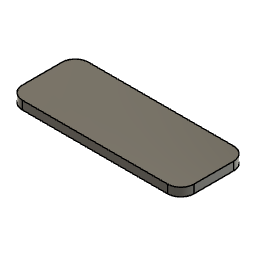
Locker Sign (Autodesk Fusion 360 design; units mm, degrees)
Autodesk Fusion 360 part; units mm, degrees
note: some values were not read from the file. Set by a fixed rule: which sketch regions a step uses.
sketch "Sketch1" plane through (0, 0, 0) normal (0, 1, 0) x (1, 0, 0)
  line L0 (30, 50) -> (140, 50)
  line L1 (150, 40) -> (150, 10)
  line L2 (140, 0) -> (30, 0)
  line L3 (20, 10) -> (20, 40)
  arc A0 (150, 40) -> (140, 50) centre (140, 40) ccw
  arc A1 (140, 0) -> (150, 10) centre (140, 10) ccw
  arc A2 (30, 50) -> (20, 40) centre (30, 40) ccw
  arc A3 (20, 10) -> (30, 0) centre (30, 10) ccw
  point P0 (20, 50)
  point P1 (150, 50)
  point P2 (20, 0)
  dimension "d1" = 130
  dimension "d2" = 50
  dimension "d7" = 10
  dimension "d8" = 10
  dimension "d9" = 10
  dimension "d10" = 10
  constraint horizontal L0
  constraint vertical L1
  constraint horizontal L2
  constraint vertical L3
  constraint coincident P1 L0
  constraint coincident P1 L1
  constraint tangent L0 A0
  constraint tangent L1 A0
  constraint tangent L1 A1
  constraint tangent L2 A1
  constraint coincident P0 L0
  constraint coincident P0 L3
  constraint tangent L0 A2
  constraint tangent L3 A2
  constraint coincident P2 L2
  constraint coincident P2 L3
  constraint tangent L2 A3
  constraint tangent L3 A3
  measures "d1" distance of P0 P1
  measures "d2" distance of P0 P2
  measures "d7" radius of A0
  measures "d8" radius of A1
  measures "d9" radius of A2
  measures "d10" radius of A3
extrude "Extrude1" add sketch "Sketch1" along normal blind 6.35
